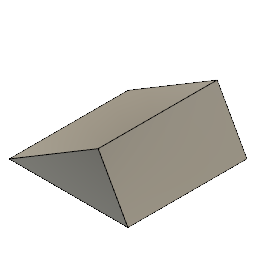
pistand (Autodesk Fusion 360 design; units mm, degrees)
Autodesk Fusion 360 part; units mm, degrees
sketch "Sketch1" plane through (0, 0, 0) normal (0, 0, 1) x (1, 0, 0)
  line L0 (0, 25) -> (25, -20)
  line L1 (25, -20) -> (-75, -20)
  line L2 (-75, -20) -> (0, 25)
  constraint horizontal L1
extrude "Extrude1" add sketch "Sketch1" along normal blind 100
move_body "Move1" bodies 1 to x (1, 0, 0) y (0, 0, 1) z (0, -1, 0) at (70, 0, 20)
